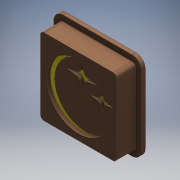
# Autodesk Inventor part: button2
Saved by Autodesk Inventor 2016 (Build 200138000, 138)
## iProperties
Created: 2017-11-06
Part Number: button2
Material: Bronze, Soft Tin
Document SubType Name: Modeling
Designer: Davide
Density: 8.874 g/cm^3
Appearance: Bronze - Satin
Author: Davide
Autodesk Inventor part; units mm, degrees
ref_plane "YZ Plane" through (0, 0, 0) normal (1, 0, 0) x (0, 1, 0)
ref_plane "XZ Plane" through (0, 0, 0) normal (0, 1, 0) x (-1, 0, 0)
ref_plane "XY Plane" through (0, 0, 0) normal (0, 0, 1) x (1, 0, 0)
sketch "Sketch1" plane through (0, 0, 0) normal (0, 1, 0) x (-1, 0, 0)
  line L0 (9, -10) -> (-9, -10)
  line L1 (-10, -9) -> (-10, 9)
  line L2 (-9, 10) -> (9, 10)
  line L3 (10, 9) -> (10, -9)
  line L4 (10, 10) -> (-10, -10) construction
  line L5 (10, -10) -> (-10, 10) construction
  arc A0 (10, 9) -> (9, 10) centre (9, 9) ccw
  arc A1 (9, -10) -> (10, -9) centre (9, -9) ccw
  arc A2 (-10, -9) -> (-9, -10) centre (-9, -9) ccw
  arc A3 (-9, 10) -> (-10, 9) centre (-9, 9) ccw
  point P0 (0, 0)
  point P1 (0, 0)
  dimension "d7" = 20
  dimension "d9" = 20
  dimension "d10" = 1
  constraints: 12 end point, 8 point on circle, 8 point on line, 8 tangent, 4 centre point, 3 equal radius, 2 parallel, 1 coincident, 1 horizontal, 1 midpoint, 1 perpendicular
  measures "d7" distance of L5.start L4.end
  measures "d9" distance of L4.end L5.end
  measures "d10" radius of A0
extrude "Extrusion1" add sketch "Sketch1" along normal blind 5
sketch "Sketch2" plane through (0, 5, 0) normal (0, 1, 0) x (1, 0, 0)
  line L0 (-10, 9) -> (-10, -9) projected
  arc A0 (-10, -9) -> (-9, -10) centre (-9, -9) ccw projected
  line L1 (-9, -10) -> (9, -10) projected
  arc A1 (9, -10) -> (10, -9) centre (9, -9) ccw projected
  line L2 (10, -9) -> (10, 9) projected
  arc A2 (10, 9) -> (9, 10) centre (9, 9) ccw projected
  line L3 (9, 10) -> (-9, 10) projected
  arc A3 (-9, 10) -> (-10, 9) centre (-9, 9) ccw projected
  line L4 (9, -11.5) -> (-9, -11.5)
  arc A4 (-11.5, -9) -> (-9, -11.5) centre (-9, -9) ccw
  line L5 (-11.5, -9) -> (-11.5, 9)
  arc A5 (-9, 11.5) -> (-11.5, 9) centre (-9, 9) ccw
  line L6 (-9, 11.5) -> (9, 11.5)
  arc A6 (11.5, 9) -> (9, 11.5) centre (9, 9) ccw
  line L7 (11.5, 9) -> (11.5, -9)
  arc A7 (9, -11.5) -> (11.5, -9) centre (9, -9) ccw
  circle A8 centre (0, 0) radius 2.75
  dimension "d16" = 1.5
  dimension "d19" = 5.5
  constraints: 8 end point, 8 point on circle, 5 centre point, 1 coincident, 7 other
  measures "d16" distance between parallel lines of L1 L4
  measures "d19" diameter of A8
extrude "Extrusion3" add sketch "Sketch2" along normal blind 1 contours A3 L3 A2 L2 A1 L1 A0 L0 | L4 A4 L5 A5 L6 A6 L7 A7
sketch "Sketch3" plane through (0, 0, 0) normal (0, -1, 0) x (1, 0, 0)
  arc A0 (-1.7009, 8.226) -> (6.2735, -5.586) centre (1.7321, 1) ccw
  arc A1 (-1.7009, 8.226) -> (6.2735, -5.586) centre (0, 0) ccw
  line L0 (0, 0) -> (1.7321, 1) construction
  circle A2 centre (0, 0) radius 2.75 construction
  line L1 (0, 0) -> (9.8042, 0) construction
  line L2 (0.8682, 8.924) -> (0.3902, 6.2132)
  line L3 (0.3902, 3.6349) -> (0.8682, 0.924)
  line L4 (0.8682, 0.924) -> (1.3462, 3.6349)
  line L5 (1.3462, 6.2132) -> (0.8682, 8.924)
  line L6 (2.1574, 4.446) -> (4.8682, 4.924)
  line L7 (4.8682, 4.924) -> (2.1574, 5.402)
  line L8 (0.8682, 8.924) -> (0.8682, 0.924) construction
  line L9 (-3.1318, 4.924) -> (4.8682, 4.924) construction
  line L10 (-0.4209, 5.402) -> (-3.1318, 4.924)
  line L11 (-3.1318, 4.924) -> (-0.4209, 4.446)
  arc A3 (-0.4209, 5.402) -> (0.3902, 6.2132) centre (-0.5946, 6.3868) ccw
  arc A4 (1.3462, 6.2132) -> (2.1574, 5.402) centre (2.331, 6.3868) ccw
  arc A5 (2.1574, 4.446) -> (1.3462, 3.6349) centre (2.331, 3.4612) ccw
  arc A6 (0.3902, 3.6349) -> (-0.4209, 4.446) centre (-0.5946, 3.4612) ccw
  line L12 (6.0644, 4.924) -> (5.7363, 3.0633)
  line L13 (5.7363, 0.7848) -> (6.0644, -1.076)
  line L14 (6.0644, -1.076) -> (6.3925, 0.7848)
  line L15 (6.3925, 3.0633) -> (6.0644, 4.924)
  line L16 (7.2037, 1.5959) -> (9.0644, 1.924)
  line L17 (9.0644, 1.924) -> (7.2037, 2.2521)
  line L18 (6.0644, 4.924) -> (6.0644, -1.076) construction
  line L19 (3.0644, 1.924) -> (9.0644, 1.924) construction
  line L20 (4.9251, 2.2521) -> (3.0644, 1.924)
  line L21 (3.0644, 1.924) -> (4.9251, 1.5959)
  arc A7 (4.9251, 2.2521) -> (5.7363, 3.0633) centre (4.7515, 3.2369) ccw
  arc A8 (6.3925, 3.0633) -> (7.2037, 2.2521) centre (7.3773, 3.2369) ccw
  arc A9 (7.2037, 1.5959) -> (6.3925, 0.7848) centre (7.3773, 0.6111) ccw
  arc A10 (5.7363, 0.7848) -> (4.9251, 1.5959) centre (4.7515, 0.6111) ccw
  line L22 (0.8682, 4.924) -> (6.0644, 1.924) construction
  line L23 (0, 0) -> (0.8682, 4.924) construction
  dimension "d37" = 2
  dimension "d41" = 16
  dimension "d42" = 16.8
  dimension "d43" = 30
  dimension "d49" = 20
  dimension "d51" = 20
  dimension "d52" = 20
  dimension "d53" = 20
  dimension "d54" = 8
  dimension "d55" = 8
  dimension "d56" = 1
  dimension "d57" = 1
  dimension "d58" = 20
  dimension "d59" = 20
  dimension "d60" = 20
  dimension "d61" = 20
  dimension "d62" = 6
  dimension "d63" = 6
  dimension "d64" = 1
  dimension "d65" = 1
  dimension "d68" = 6
  dimension "d69" = 80
  dimension "d70" = 70
  dimension "d71" = 5
  constraints: 48 end point, 20 point on circle, 16 tangent, 10 centre point, 4 equal radius, 4 midpoint, 2 coincident, 2 parallel, 2 perpendicular, 2 point on line, 1 horizontal, 8 other
  measures "d37" distance of L0.start L0.end
  measures "d41" diameter of A0
  measures "d42" diameter of A1
  measures "d43" angle of L1 L0
  measures "d49" angle of L5 L2
  measures "d51" angle of L6 L7
  measures "d52" angle of L4 L3
  measures "d53" angle of L10 L11
  measures "d54" distance of L2.start L8.end
  measures "d55" distance of L9.start L6.end
  measures "d56" radius of A3
  measures "d57" radius of A4
  measures "d58" angle of L15 L12
  measures "d59" angle of L16 L17
  measures "d60" angle of L14 L13
  measures "d61" angle of L20 L21
  measures "d62" distance of L18.start L18.end
  measures "d63" distance of L20.end L16.end
  measures "d64" radius of A7
  measures "d65" radius of A8
  measures "d68" distance of L22.start L22.end
  measures "d69" angle of L1 L23
  measures "d70" angle of L22 L23
  measures "d71" distance of L1.start L22.start
extrude "Extrusion5" cut sketch "Sketch3" against normal blind 1
hole "Hole1" at (0, 5, 0) direction (0, -1, 0) diameter 5.5 depth 3
equation "\"d7\" = button_side"
equation "\"d9\" = d7"
equation "\"d37\" = 0.1 * button_side"
equation "\"d41\" = 0.8 * button_side"
equation "\"d42\" = 1.05 * d41"
equation "\"d51\" = d49"
equation "\"d52\" = d49"
equation "\"d53\" = d49"
equation "\"d54\" = 0.4 * button_side"
equation "\"d55\" = d54"
equation "\"d59\" = d58"
equation "\"d60\" = d58"
equation "\"d61\" = d58"
equation "\"d62\" = 0.3 * button_side"
equation "\"d63\" = d62"
equation "\"d68\" = 0.3 * button_side"
equation "\"d0\" = 122"
equation "\"d1\" = 77"
equation "\"d4\" = 19"
equation "\"d5\" = 1"
equation "\"d8\" = 25"
equation "\"d13\" = 1.5"
equation "\"d14\" = 0"
equation "\"d15\" = 2"
equation "\"d30\" = 3.1"
equation "\"d31\" = 3"
equation "\"d33\" = 3"
equation "\"d34\" = 2"
equation "\"d36\" = 3"
equation "\"d38\" = 90deg"
equation "\"d39\" = 8"
equation "\"d40\" = 118deg"
equation "\"d44\" = 0"
equation "\"d45\" = 1.2"
equation "\"d46\" = 2"
equation "\"d47\" = 0"
equation "\"d50\" = 25"
equation "\"button_side\" = 20"
equation "\"d3\" = 1.01 * button_side"
equation "\"d2\" = d3"
body "Solid1"
